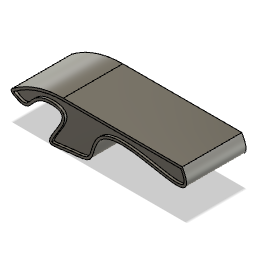
BottleOpener_09102021_2049 (Autodesk Fusion 360 design; units mm, degrees)
Autodesk Fusion 360 part; units mm, degrees
sketch "Sketch1" plane through (0, 0, 0) normal (0, 0, 1) x (1, 0, 0)
  line L0 (35.1167, 35.0496) -> (-14.8833, 35.0496)
  arc A0 (-14.8833, 35.0496) -> (-37.3847, 26.9894) centre (-14.8833, -0.3887) ccw
  spline S0 degree 5 poles (-37.3847, 26.9894) (-37.0794, 26.7566) (-36.4115, 26.2745) (-35.2377, 25.5016) (-33.4233, 24.5135) (-31.1851, 24) (-29.3394, 24.693) (-27.9367, 26.5467) (-26.3115, 28.3486) (-24.2671, 29.6332) (-21.85, 30.2653) (-19.3243, 30.3431) (-17.069, 30.0039) (-15.5178, 29.2246) (-15.0455, 27.797) (-15.8059, 25.5739) (-17.5788, 22.6482) (-19.6141, 19.5565) (-20.9396, 17.0257) (-20.7877, 15.6011) (-18.7754, 15.5282) (-15.6683, 16.0299) (-12.3187, 16.4817) (-9.1971, 16.7912) (-6.6234, 17.062) (-4.7101, 17.5486) (-3.4297, 18.4961) (-2.6251, 20.0082) (-2.0517, 21.9723) (-1.4259, 24.1594) (-0.4759, 26.2873) (1.0125, 28.0933) (3.1376, 29.415) (5.8882, 30.1944) (9.1729, 30.4506) (12.8416, 30.2639) (16.7102, 29.7545) (20.5841, 29.0644) (24.2808, 28.3382) (27.6561, 27.7026) (30.6032, 27.2636) (33.0454, 27.1091) (34.931, 27.3088) (36.2277, 27.9155) (36.9171, 28.9654) (36.9895, 30.4794) (36.5508, 32.0695) (35.9424, 33.4763) (35.4126, 34.5093) (35.1167, 35.0496) knots 0 0 0 0 0 0 0.022222 0.044444 0.066667 0.088889 0.111111 0.133333 0.155556 0.177778 0.2 0.222222 0.244444 0.266667 0.288889 0.311111 0.333333 0.355556 0.377778 0.4 0.422222 0.444444 0.466667 0.488889 0.511111 0.533333 0.555556 0.577778 0.6 0.622222 0.644444 0.666667 0.688889 0.711111 0.733333 0.755556 0.777778 0.8 0.822222 0.844444 0.866667 0.888889 0.911111 0.933333 0.955556 0.977778 1 1 1 1 1 1
  line L1 (-24.9932, 15.5713) -> (-12.9029, 15.7392)
  line L2 (-43.2215, 31.4393) -> (-31.5479, 22.5395)
  line L3 (-33.8988, 20.2725) -> (-23.4877, 31.0195)
  point P0 (-28.6933, 25.646)
  point P1 (-18.1142, 30.0959)
  point P2 (-16.0992, 25.3102)
  point P3 (-18.9481, 15.6552)
  point P4 (-3.9249, 18.2575)
  point P5 (0.0212, 26.7375)
  point P6 (36.0403, 27.9969)
  point P7 (21.2632, 28.9205)
  dimension "d1" = 50
  constraint horizontal L0
  constraint tangent L0 A0
  constraint midpoint P3 L1
  constraint midpoint A0.end L2
  constraint midpoint P0 L3
  measures "d1" distance of L0.start L0.end
extrude "Extrude1" add sketch "Sketch1" along normal blind 25 contours L0 A0 S0
ref_plane "WorkPlane1" through (-0.243, 25.3452, 12.5) normal (0, 0, 1) x (1, 0, 0)
sketch "Sketch2" plane through (-0.2377, 25.2595, 12.5) normal (0, 0, 1) x (1, 0, 0)
  line L0 (-22.9304, -4.7902) -> (-4.9304, -4.7902)
  line L1 (-4.9304, -4.7902) -> (-4.9304, -6.1902)
  line L2 (-4.9304, -6.1902) -> (-22.9304, -6.1902)
  line L3 (-22.9304, -6.1902) -> (-22.9304, -4.7902)
  line L4 (-19.9304, -4.7902) -> (-19.9304, -6.1902) construction
  dimension "d4" = 18
  dimension "d5" = 1.4
  dimension "d6" = 3
  constraint horizontal L0
  constraint vertical L1
  constraint horizontal L2
  constraint vertical L3
  constraint coincident L0 L4.start
  constraint coincident L2 L4.end
  constraint perpendicular L2 L4
  measures "d4" distance of L0.start L0.end
  measures "d5" distance of L0.start L2.end
  measures "d6" distance of L3 L4.start
extrude "Extrude2" cut sketch "Sketch2" along normal mid plane 18
sketch "Sketch3" plane through (0, 0, 25) normal (0, 0, 1) x (1, 0, 0)
  spline S0 degree 5 poles (-37.3847, 26.9894) (-37.0794, 26.7566) (-36.4115, 26.2745) (-35.2377, 25.5016) (-33.4233, 24.5135) (-31.1851, 24) (-29.3394, 24.693) (-27.9367, 26.5467) (-26.3115, 28.3486) (-24.2671, 29.6332) (-21.85, 30.2653) (-19.3243, 30.3431) (-17.069, 30.0039) (-15.5178, 29.2246) (-15.0455, 27.797) (-15.8059, 25.5739) (-17.5788, 22.6482) (-19.6141, 19.5565) (-20.9396, 17.0257) (-20.7877, 15.6011) (-18.7754, 15.5282) (-15.6683, 16.0299) (-12.3187, 16.4817) (-9.1971, 16.7912) (-6.6234, 17.062) (-4.7101, 17.5486) (-3.4297, 18.4961) (-2.6251, 20.0082) (-2.0517, 21.9723) (-1.4259, 24.1594) (-0.4759, 26.2873) (1.0125, 28.0933) (3.1376, 29.415) (5.8882, 30.1944) (9.1729, 30.4506) (12.8416, 30.2639) (16.7102, 29.7545) (20.5841, 29.0644) (24.2808, 28.3382) (27.6561, 27.7026) (30.6032, 27.2636) (33.0454, 27.1091) (34.931, 27.3088) (36.2277, 27.9155) (36.9171, 28.9654) (36.9895, 30.4794) (36.5508, 32.0695) (35.9424, 33.4763) (35.4126, 34.5093) (35.1167, 35.0496) knots 0 0 0 0 0 0 0.022222 0.044444 0.066667 0.088889 0.111111 0.133333 0.155556 0.177778 0.2 0.222222 0.244444 0.266667 0.288889 0.311111 0.333333 0.355556 0.377778 0.4 0.422222 0.444444 0.466667 0.488889 0.511111 0.533333 0.555556 0.577778 0.6 0.622222 0.644444 0.666667 0.688889 0.711111 0.733333 0.755556 0.777778 0.8 0.822222 0.844444 0.866667 0.888889 0.911111 0.933333 0.955556 0.977778 1 1 1 1 1 1
  line L0 (35.1167, 35.0496) -> (-14.8833, 35.0496)
  arc A0 (-14.8833, 35.0496) -> (-37.3847, 26.9894) centre (-14.8833, -0.3887) ccw
  spline S1 degree 3 poles (-35.7172, 27.0329) (-35.0799, 26.612) (-34.3589, 26.1868) (-33.6466, 25.8639) (-32.7831, 25.4725) (-31.9564, 25.2612) (-31.328, 25.2961) (-30.6556, 25.3335) (-30.1631, 25.5965) (-29.5365, 26.2154) (-28.8148, 26.9283) (-27.9745, 28.0481) (-26.9061, 28.9427) (-25.7953, 29.8728) (-24.4274, 30.5676) (-22.9785, 30.9198) (-21.2888, 31.3306) (-19.5172, 31.3486) (-17.9923, 31.0896) (-17.0389, 30.9277) (-16.166, 30.667) (-15.4535, 30.1144) (-14.9297, 29.7081) (-14.5216, 29.0927) (-14.3939, 28.4009) (-14.2038, 27.3703) (-14.533, 26.2895) (-15.0909, 25.1001) (-15.7604, 23.6729) (-16.825, 22.0361) (-17.7795, 20.5022) (-18.3845, 19.53) (-18.9343, 18.6083) (-19.2763, 17.8838) (-19.5349, 17.3362) (-19.6591, 16.8925) (-19.6703, 16.7143) knots 0.01452 0.01452 0.01452 0.01452 0.038134 0.038134 0.038134 0.066756 0.066756 0.066756 0.097383 0.097383 0.097383 0.132663 0.132663 0.132663 0.169344 0.169344 0.169344 0.212121 0.212121 0.212121 0.238864 0.238864 0.238864 0.258525 0.258525 0.258525 0.287812 0.287812 0.287812 0.322952 0.322952 0.322952 0.345226 0.345226 0.345226 0.36206 0.36206 0.36206 0.36206
  spline S2 degree 3 poles (-19.6703, 16.7143) (-19.5654, 16.685) (-19.358, 16.6567) (-19.0814, 16.6547) (-18.2255, 16.6485) (-16.7762, 16.868) (-15.2774, 17.0776) (-13.3681, 17.3446) (-11.3514, 17.5725) (-9.6572, 17.7536) (-8.0359, 17.9269) (-6.7073, 18.0889) (-5.815, 18.3706) (-4.9214, 18.6527) (-4.469, 18.9925) (-4.0603, 19.6154) (-3.6079, 20.305) (-3.2674, 21.4311) (-2.8603, 22.7638) (-2.3533, 24.423) (-1.6802, 26.3655) (-0.3124, 27.9119) (0.8705, 29.2492) (2.5526, 30.2393) (4.5866, 30.7755) (7.7037, 31.5974) (11.6664, 31.4209) (15.7113, 30.865) (19.8151, 30.3011) (23.9365, 29.3898) (27.2817, 28.8116) (29.6331, 28.4052) (31.6196, 28.1622) (33.0545, 28.2006) (34.1694, 28.2305) (34.9257, 28.4419) (35.3143, 28.7032) (35.6186, 28.9079) (35.7549, 29.1049) (35.8361, 29.4927) (35.9544, 30.0574) (35.8236, 31.0834) (35.2507, 32.483) (35.0542, 32.9633) (34.8097, 33.4864) (34.5171, 34.0496) knots 0.384436 0.384436 0.384436 0.384436 0.394455 0.394455 0.394455 0.425462 0.425462 0.425462 0.464962 0.464962 0.464962 0.502762 0.502762 0.502762 0.540619 0.540619 0.540619 0.582532 0.582532 0.582532 0.634715 0.634715 0.634715 0.679842 0.679842 0.679842 0.748999 0.748999 0.748999 0.819164 0.819164 0.819164 0.868484 0.868484 0.868484 0.906805 0.906805 0.906805 0.93681 0.93681 0.93681 0.980496 0.980496 0.980496 0.995486 0.995486 0.995486 0.995486
  line L1 (34.5171, 34.0496) -> (-14.8833, 34.0496)
  arc A1 (-14.8833, 34.0496) -> (-35.7172, 27.0329) centre (-14.8833, -0.3887) ccw
  dimension "d9" = -1
extrude "Extrude3" cut sketch "Sketch3" against normal blind 1 contours S1 S2 L1 A1
mirror "Mirror1" about plane through (-0.243, 25.3452, 12.5) normal (0, 0, 1) of "Extrude3"
fillet "Fillet1" radius 1 1 edges at (-37.3847, 26.9894, 12.5)
